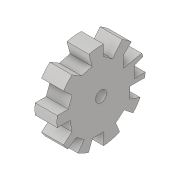
# Autodesk Inventor part: pinion
Saved by Autodesk Inventor 2019 (Build 230136000, 136)
## iProperties
Created: 2020-02-12
Part Number: pinion
Material: Generic
Document SubType Name: Modeling
Designer: Admin
Density: 1 g/cm^3
Appearance: Default
Author: Admin
Autodesk Inventor part; units mm, degrees
ref_plane "YZ Plane" through (0, 0, 0) normal (1, 0, 0) x (0, 1, 0)
ref_plane "XZ Plane" through (0, 0, 0) normal (0, 1, 0) x (-1, 0, 0)
ref_plane "XY Plane" through (0, 0, 0) normal (0, 0, 1) x (1, 0, 0)
sketch "Sketch1" plane through (0, 0, 0) normal (1, 0, 0) x (0, 1, 0)
  circle A0 centre (0, 0) radius 40
  dimension "d0" = 80
  constraints: 1 centre point, 1 coincident
  measures "d0" diameter of A0
extrude "Extrusion1" add sketch "Sketch1" along normal blind 20
sketch "Sketch2" plane through (20, 0, 0) normal (1, 0, 0) x (0, 0, -1)
  circle A0 centre (0, 0) radius 40 projected
  line L0 (-11.3165, -38.3658) -> (-7.7264, -29.0325)
  line L1 (-7.7264, -29.0325) -> (2.2736, -29.0325)
  line L2 (2.2736, -29.0325) -> (2.2736, -39.9353)
  line L3 (16.8851, -36.2615) -> (13.3323, -27.4978)
  line L4 (13.3323, -27.4978) -> (20.9893, -21.0659)
  line L5 (20.9893, -21.0659) -> (29.0495, -27.4978)
  line L6 (-34.0034, -21.0659) -> (-26.3463, -14.6339)
  line L7 (-26.3463, -14.6339) -> (-28.141, -4.7963)
  line L8 (-28.141, -4.7963) -> (-39.7114, -4.7963)
  line L9 (-39.7114, 4.7963) -> (-29.7114, 4.7963)
  line L10 (-29.7114, 4.7963) -> (-26.3463, 14.2131)
  line L11 (-26.3463, 14.2131) -> (-33.9262, 21.1899)
  line L12 (35.4673, -18.4951) -> (26.0505, -15.1301)
  line L13 (26.0505, -15.1301) -> (26.0505, -5.1301)
  line L14 (26.0505, -5.1301) -> (39.6697, -5.1301)
  line L15 (-26.3463, 30.0977) -> (-17.7279, 25.026)
  line L16 (-17.7279, 25.026) -> (-8.0547, 27.5618)
  line L17 (-8.0547, 27.5618) -> (-10.9173, 38.4813)
  line L18 (2.2736, 39.9353) -> (2.2736, 30.2694)
  line L19 (2.2736, 30.2694) -> (10.2947, 24.2977)
  line L20 (10.2947, 24.2977) -> (19.1787, 35.1024)
  line L21 (27.4627, 29.0827) -> (20.2021, 22.2063)
  line L22 (20.2021, 22.2063) -> (20.2021, 12.2063)
  line L23 (20.2021, 12.2063) -> (36.9402, 15.3435)
  line L24 (39.9893, -0.9244) -> (29.9893, -0.9244)
  line L25 (29.9893, -0.9244) -> (30.7589, 9.5047)
  line L26 (30.7589, 9.5047) -> (38.0921, 12.2063)
  dimension "d3" = 10
  dimension "d4" = 10
  dimension "d5" = 10
  dimension "d6" = 10
  dimension "d7" = 10
  dimension "d8" = 10
  dimension "d9" = 10
  dimension "d10" = 10
  dimension "d11" = 10
  dimension "d12" = 10
  dimension "d13" = 10
  dimension "d14" = 10
  dimension "d15" = 10
  dimension "d16" = 10
  dimension "d17" = 10
  constraints: 54 end point, 4 horizontal, 3 perpendicular, 3 vertical, 19 other
  measures "d3" distance of L0.start L0.end
  measures "d4" distance of L0.end L1.end
  measures "d5" distance of L3.end L4.end
  measures "d6" distance of L6.start L6.end
  measures "d7" distance of L6.end L7.end
  measures "d8" distance of L9.start L9.end
  measures "d9" distance of L9.end L10.end
  measures "d10" distance of L12.start L12.end
  measures "d11" distance of L12.end L13.end
  measures "d12" distance of L15.start L15.end
  measures "d13" distance of L15.end L16.end
  measures "d14" distance of L18.end L19.end
  measures "d15" distance of L21.start L21.end
  measures "d16" distance of L21.end L22.end
  measures "d17" distance of L24.start L24.end
extrude "Extrusion2" cut sketch "Sketch2" against normal blind 20 contours A0 L24 L25 L26 | L23 L22 L21 A0 | A0 L12 L13 L14 | L20 L19 L18 A0 | A0 L3 L4 L5 | L17 L16 L15 A0 | A0 L0 L1 L2 | L11 L10 L9 A0 | A0 L8 L7 L6
sketch "Sketch3" plane through (20, 0, 0) normal (1, 0, 0) x (0, 0, -1)
  arc A0 (-34.0034, -21.0659) -> (-11.3165, -38.3658) centre (0, 0) ccw projected
  line L0 (-30.137, -26.3014) -> (-22.2204, -21.0659)
  line L1 (-22.2204, -21.0659) -> (-15.2765, -26.3014)
  line L2 (-15.2765, -26.3014) -> (-21.078, -33.9959)
  constraints: 6 end point, 2 point on circle, 1 perpendicular
extrude "Extrusion3" cut sketch "Sketch3" against normal blind 20
sketch "Sketch4" plane through (20, 0, 0) normal (1, 0, 0) x (0, 0, -1)
  circle A0 centre (0, 0) radius 5
  dimension "d22" = 10
  constraints: 1 centre point, 1 coincident
  measures "d22" diameter of A0
extrude "Extrusion4" cut sketch "Sketch4" against normal blind 20
body "Solid1"
